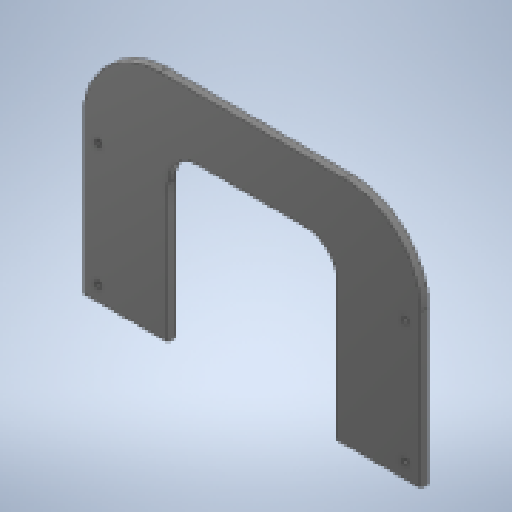
# Autodesk Inventor part: speaker_front
Saved by Autodesk Inventor 2026.2 (Build 302298010, 298A)
## iProperties
Created: 2026-05-31
Part Number: speaker_front
Material: ABS Plastic
Document SubType Name: Modeling
Designer: chris
Density: 1.06 g/cm^3
Appearance: Smooth - White
Author: chris
Autodesk Inventor part; units mm, degrees
ref_plane "YZ Plane" through (0, 0, 0) normal (1, 0, 0) x (0, 1, 0)
ref_plane "XZ Plane" through (0, 0, 0) normal (0, 1, 0) x (-1, 0, 0)
ref_plane "XY Plane" through (0, 0, 0) normal (0, 0, 1) x (1, 0, 0)
sketch "Sketch1" plane through (0, 0, 0) normal (0, 0, 1) x (1, 0, 0)
  line L0 (-110, -75) -> (110, -75)
  line L1 (110, -75) -> (110, 75)
  line L2 (110, 75) -> (-110, 75)
  line L3 (-110, 75) -> (-110, -75)
  line L4 (-110, -75) -> (110, 75) construction
  line L5 (110, -75) -> (-110, 75) construction
  point P0 (0, 0)
  dimension "d0" = 220
  dimension "d1" = 150
  constraints: 12 end point, 2 midpoint, 2 parallel, 1 horizontal, 1 perpendicular
  measures "d0" distance of L2.end L1.end
  measures "d1" distance of L1.end L0.end
extrude "Extrusion1" add sketch "Sketch1" along normal blind 5
sketch "Sketch2" plane through (0, 0, 0) normal (0, 0, -1) x (-1, 0, 0)
  circle A0 centre (100, 15) radius 2 projected
  circle A1 centre (-100, -65) radius 2 projected
  circle A2 centre (100, -65) radius 2 projected
  circle A3 centre (-100, 15) radius 2 projected
  line L0 (-110, -75) -> (-80, -75) projected
  line L1 (-80, -75) -> (-80, -70) projected
  line L2 (-95, -70) -> (-80, -70) projected
  line L3 (-95, -70) -> (-95, -60) projected
  line L4 (-95, -60) -> (-105, -60) projected
  line L5 (-105, -60) -> (-105, 10) projected
  line L6 (-105, 10) -> (-95, 10) projected
  line L7 (-95, 10) -> (-95, 20) projected
  line L8 (-95, 20) -> (-105, 20) projected
  line L9 (-105, 20) -> (-105, 25) projected
  arc A4 (-60, 70) -> (-105, 25) centre (-60, 25) ccw projected
  line L10 (-60, 70) -> (60, 70) projected
  arc A5 (105, 25) -> (60, 70) centre (60, 25) ccw projected
  line L11 (105, 20) -> (105, 25) projected
  line L12 (105, 20) -> (95, 20) projected
  line L13 (95, 20) -> (95, 10) projected
  line L14 (95, 10) -> (105, 10) projected
  line L15 (105, -60) -> (105, 10) projected
  line L16 (105, -60) -> (95, -60) projected
  line L17 (95, -60) -> (95, -70) projected
  line L18 (80, -70) -> (95, -70) projected
  line L19 (80, -70) -> (80, -75) projected
  line L20 (80, -75) -> (110, -75) projected
  line L21 (110, -75) -> (110, 25) projected
  arc A6 (110, 25) -> (60, 75) centre (60, 25) ccw projected
  line L22 (-60, 75) -> (60, 75) projected
  arc A7 (-60, 75) -> (-110, 25) centre (-60, 25) ccw projected
  line L23 (-110, -75) -> (-110, 25) projected
  line L24 (-110, -75) -> (110, -75)
  line L25 (110, -75) -> (110, 75)
  line L26 (110, 75) -> (-110, 75)
  line L27 (-110, 75) -> (-110, -75)
  line L28 (-110, -75) -> (110, 75) construction
  line L29 (110, -75) -> (-110, 75) construction
  point P0 (0, 0)
  point P1 (-110, 25)
  constraints: 12 end point, 2 midpoint, 2 parallel, 1 horizontal, 1 perpendicular
extrude "Extrusion2" cut sketch "Sketch2" against normal blind 5 contours A0 | A1 | A2 | A3 | L27 L26 A7 | L26 L25 A6
sketch "Sketch4" plane through (0, 0, 0) normal (0, 0, -1) x (-1, 0, 0)
  line L0 (-55, -75) -> (55, -75)
  line L1 (55, -75) -> (55, 15)
  line L2 (35, 35) -> (-35, 35)
  line L3 (-55, 15) -> (-55, -75)
  line L4 (110, -75) -> (-110, -75) projected
  arc A0 (-35, 35) -> (-55, 15) centre (-35, 15) ccw
  arc A1 (55, 15) -> (35, 35) centre (35, 15) ccw
  point P0 (0, 0)
  point P1 (55, 35)
  point P2 (-55, 35)
  dimension "d12" = 110
  dimension "d13" = 110
  dimension "d14" = 55
  dimension "d15" = 20
  constraints: 8 end point, 4 point on circle, 4 point on line, 4 tangent, 2 centre point, 2 parallel, 1 collinear, 1 equal radius, 1 horizontal, 1 perpendicular
  measures "d12" distance of point (-55, 35) point (55, 35)
  measures "d13" distance of point (55, 35) L0.end
  measures "d14" distance from line of L1 point (0, 0)
  measures "d15" radius of A0
extrude "Extrusion4" cut sketch "Sketch4" against normal blind 5
body "Solid1"
